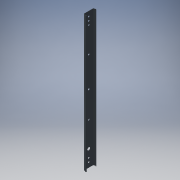
# Autodesk Inventor part: body_SSRN3618
Saved by Autodesk Inventor 2016 (Build 200138000, 138)
## iProperties
Category: PARTsolutions
Company: MISUMI
Created: 2016-11-23
Part Number: body_SSRN3618
Catalog Web Link: www.cadenas.de
Description: body_ssrn36-Slide Rails - Stainles Steel - Two - Step Slide Rails
Vendor: MISUMI
Document SubType Name: Modeling
Designer: psAdmin
Manufacturer: MISUMI
Mass: 83.9848 g
Surface Area: 460.954 cm^2
Volume: 11.7461 cm^3
Density: 7.15 g/cm^3
Material: 鉄 灰色
Appearance: 鉄 灰色
PSOL_IDENT_0: {$CADENAS_DATA\23d-libs\misumi\metric\07_slide_rails\ssrn36_series\ssrn36_body.prj},166 {VTYP=3D},{N
PSOL_IDENT_1: B=body_SSRN3618},{LINA=body_SSRN3618},{NN=body_ssrn36},{DATE=17.06.2016 05:46:12},{GEOMDATE=16.03.20
PSOL_IDENT_2: 05},{VERSION=},{LINEID=10},{LINESUBID=-1},{WBVAR=NO}  {NB=body_SSRN3618},{LINA=body_SSRN3618},{KT=DU
PSOL_IDENT_3: MMY},{PN=SSRN3618},{TYPE=SSRN3618},{MATR=Rail 304 Stainless Steel},{MATB=Ball 440C Stainless Steel},
PSOL_IDENT_4: {NO=18},{RL=457.2},{TD=330.2},{A=203.2},{B=304.8},{C=406.4},{D=212.7},{E=301.6},{F=412.7},{G=425.4},
PSOL_IDENT_5: {RLD=402}
NN: body_ssrn36
NT: Slide Rails - Stainles Steel - Two - Step Slide Rails
NB: body_SSRN3618
NBSYN: body_$PN.
LINA: body_SSRN3618
MATR: Rail 304 Stainless Steel
MATB: Ball 440C Stainless Steel
NO: 18
SUPPLIER: MISUMI
ARTICLENO: body_SSRN3618
BOMINFO: body_SSRN3618
CREATOR: CADENAS GmbH
Title: body_SSRN3618
Author: Cadenas PARTsolutions
Comments: Slide Rails - Stainles Steel - Two - Step Slide Rails
Autodesk Inventor part; units mm, degrees
sketch "Sketch_1" plane through (0, 0, 0) normal (0, 0, 1) x (1, 0, 0)
  line L0 (0, 32.8967) -> (0, 2.4033)
  line L1 (0, 2.4033) -> (6.2112, 0)
  line L2 (6.2112, 0) -> (7.15, 0)
  arc A0 (7.15, 0) -> (9, 1.85) centre (7.15, 1.85) ccw
  line L3 (9, 1.85) -> (9, 2.1444)
  line L4 (9, 2.1444) -> (8.493, 2.1888)
  arc A1 (5.9824, 0.6246) -> (8.493, 2.1888) centre (6.65, 2.35) ccw
  line L5 (5.9824, 0.6246) -> (0.5, 2.7459)
  line L6 (0.5, 2.7459) -> (0.5, 32.5541)
  line L7 (0.5, 32.5541) -> (5.9824, 34.6754)
  arc A2 (8.493, 33.1112) -> (5.9824, 34.6754) centre (6.65, 32.95) ccw
  line L8 (8.493, 33.1112) -> (9, 33.1556)
  line L9 (9, 33.1556) -> (9, 33.45)
  arc A3 (9, 33.45) -> (7.15, 35.3) centre (7.15, 33.45) ccw
  line L10 (7.15, 35.3) -> (6.2112, 35.3)
  line L11 (6.2112, 35.3) -> (0, 32.8967)
  constraints: 24 end point, 8 point on circle, 4 centre point
extrude "Extrusion1" add sketch "Sketch_1" along normal blind 457.2
sketch "Sketch_4" plane through (0, 0, 0) normal (1, 0, 0) x (0, 1, 0)
  arc A0 (17.65, 332.85) -> (15.4, 330.6) centre (17.65, 330.6) ccw
  line L0 (15.4, 330.6) -> (15.4, 329.8)
  arc A1 (15.4, 329.8) -> (17.65, 327.55) centre (17.65, 329.8) ccw
  arc A2 (17.65, 327.55) -> (19.9, 329.8) centre (17.65, 329.8) ccw
  line L1 (19.9, 329.8) -> (19.9, 330.6)
  arc A3 (19.9, 330.6) -> (17.65, 332.85) centre (17.65, 330.6) ccw
  constraints: 8 point on circle, 4 centre point, 4 end point
extrude "Extrusion2" cut sketch "Sketch_4" along normal blind 0.5
sketch "Sketch_5" plane through (0, 0, 0) normal (1, 0, 0) x (0, 1, 0)
  arc A0 (17.65, 231.25) -> (15.4, 229) centre (17.65, 229) ccw
  line L0 (15.4, 229) -> (15.4, 228.2)
  arc A1 (15.4, 228.2) -> (17.65, 225.95) centre (17.65, 228.2) ccw
  arc A2 (17.65, 225.95) -> (19.9, 228.2) centre (17.65, 228.2) ccw
  line L1 (19.9, 228.2) -> (19.9, 229)
  arc A3 (19.9, 229) -> (17.65, 231.25) centre (17.65, 229) ccw
  constraints: 8 point on circle, 4 centre point, 4 end point
extrude "Extrusion3" cut sketch "Sketch_5" along normal blind 0.5
sketch "Sketch_6" plane through (0, 0, 0) normal (1, 0, 0) x (0, 1, 0)
  arc A0 (17.65, 142.35) -> (15.4, 140.1) centre (17.65, 140.1) ccw
  line L0 (15.4, 140.1) -> (15.4, 139.3)
  arc A1 (15.4, 139.3) -> (17.65, 137.05) centre (17.65, 139.3) ccw
  arc A2 (17.65, 137.05) -> (19.9, 139.3) centre (17.65, 139.3) ccw
  line L1 (19.9, 139.3) -> (19.9, 140.1)
  arc A3 (19.9, 140.1) -> (17.65, 142.35) centre (17.65, 140.1) ccw
  constraints: 8 point on circle, 4 centre point, 4 end point
extrude "Extrusion4" cut sketch "Sketch_6" along normal blind 0.5
sketch "Sketch_7" plane through (0, 0, 0) normal (1, 0, 0) x (0, 1, 0)
  line L0 (18.05, 443.55) -> (17.25, 443.55)
  arc A0 (17.25, 443.55) -> (15, 441.3) centre (17.25, 441.3) ccw
  arc A1 (15, 441.3) -> (17.25, 439.05) centre (17.25, 441.3) ccw
  line L1 (17.25, 439.05) -> (18.05, 439.05)
  arc A2 (18.05, 439.05) -> (20.3, 441.3) centre (18.05, 441.3) ccw
  arc A3 (20.3, 441.3) -> (18.05, 443.55) centre (18.05, 441.3) ccw
  constraints: 8 point on circle, 4 centre point, 4 end point
extrude "Extrusion5" cut sketch "Sketch_7" along normal blind 0.5
sketch "Sketch_3" plane through (0, 0, 0) normal (1, 0, 0) x (0, 1, 0)
  line L0 (18.05, 30.85) -> (17.25, 30.85)
  arc A0 (17.25, 30.85) -> (15, 28.6) centre (17.25, 28.6) ccw
  arc A1 (15, 28.6) -> (17.25, 26.35) centre (17.25, 28.6) ccw
  line L1 (17.25, 26.35) -> (18.05, 26.35)
  arc A2 (18.05, 26.35) -> (20.3, 28.6) centre (18.05, 28.6) ccw
  arc A3 (20.3, 28.6) -> (18.05, 30.85) centre (18.05, 28.6) ccw
  constraints: 8 point on circle, 4 centre point, 4 end point
extrude "Extrusion6" cut sketch "Sketch_3" along normal blind 0.5
sketch "Sketch_8" plane through (0, 0, 0) normal (1, 0, 0) x (0, 1, 0)
  line L0 (18.05, 18.15) -> (17.25, 18.15)
  arc A0 (17.25, 18.15) -> (15, 15.9) centre (17.25, 15.9) ccw
  arc A1 (15, 15.9) -> (17.25, 13.65) centre (17.25, 15.9) ccw
  line L1 (17.25, 13.65) -> (18.05, 13.65)
  arc A2 (18.05, 13.65) -> (20.3, 15.9) centre (18.05, 15.9) ccw
  arc A3 (20.3, 15.9) -> (18.05, 18.15) centre (18.05, 15.9) ccw
  constraints: 8 point on circle, 4 centre point, 4 end point
extrude "Extrusion7" cut sketch "Sketch_8" along normal blind 0.5
sketch "Sketch_9" plane through (0, 0, 0) normal (1, 0, 0) x (0, 1, 0)
  line L0 (18.05, 430.85) -> (17.25, 430.85)
  arc A0 (17.25, 430.85) -> (15, 428.6) centre (17.25, 428.6) ccw
  arc A1 (15, 428.6) -> (17.25, 426.35) centre (17.25, 428.6) ccw
  line L1 (17.25, 426.35) -> (18.05, 426.35)
  arc A2 (18.05, 426.35) -> (20.3, 428.6) centre (18.05, 428.6) ccw
  arc A3 (20.3, 428.6) -> (18.05, 430.85) centre (18.05, 428.6) ccw
  constraints: 8 point on circle, 4 centre point, 4 end point
extrude "Extrusion8" cut sketch "Sketch_9" along normal blind 0.5
sketch "Sketch_10" plane through (0, 0, 0) normal (1, 0, 0) x (0, 1, 0)
  arc A0 (17.75, 418.55) -> (15.5, 416.3) centre (17.75, 416.3) ccw
  line L0 (15.5, 416.3) -> (15.5, 415.5)
  arc A1 (15.5, 415.5) -> (17.75, 413.25) centre (17.75, 415.5) ccw
  arc A2 (17.75, 413.25) -> (20, 415.5) centre (17.75, 415.5) ccw
  line L1 (20, 415.5) -> (20, 416.3)
  arc A3 (20, 416.3) -> (17.75, 418.55) centre (17.75, 416.3) ccw
  constraints: 8 point on circle, 4 centre point, 4 end point
extrude "Extrusion9" cut sketch "Sketch_10" along normal blind 0.5
sketch "Sketch10" plane through (0, 2.4033, 0) normal (-1, 0, 0) x (0, 0, 1)
  point P0 (55, 15.2467)
hole "Hole1" at (0, 17.65, 55) direction (1, 0, 0) diameter 9.5 depth 0.5
ref_plane "to_rail_XY" through (9.5, 17.65, 228.6) normal (0, 0, 1) x (1, 0, 0)
ref_plane "to_rail_YZ" through (9.5, 17.65, 228.6) normal (1, 0, 0) x (0, 1, 0)
ref_plane "to_rail_ZX" through (9.5, 17.65, 228.6) normal (0, 1, 0) x (0, 0, 1)
body "Solid1"
